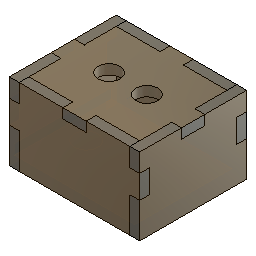
Wooden Preamp Box v5 (Autodesk Fusion 360 design; units mm, degrees)
Autodesk Fusion 360 part; units mm, degrees
note: some values were not read from the file. Chosen so that the rebuilt part matches the saved one: which face or edge a step refers to; a direction.
sketch "Sketch1" plane through (0, 0, 0) normal (1, 0, 0) x (0, 0, -1) in component "Open End"
  line L0 (-29.1465, 0) -> (-29.1465, 19.1516)
  line L1 (-29.1465, 19.1516) -> (-23.8125, 19.1516)
  line L2 (-23.8125, 19.1516) -> (-23.8125, 31.8516)
  line L3 (-23.8125, 31.8516) -> (-29.1465, 31.8516)
  line L4 (-29.1465, 31.8516) -> (-29.1465, 41.9608)
  line L5 (-29.1465, 41.9608) -> (-6.35, 41.9608)
  line L6 (-6.35, 41.9608) -> (-6.35, 36.6268)
  line L7 (-6.35, 36.6268) -> (0, 36.6268)
  line L8 (0, 36.6268) -> (0, 0)
  line L9 (-29.1465, 0) -> (-23.8125, 0)
  line L10 (-23.8125, 0) -> (-23.8125, 3.6576)
  line L11 (-23.8125, 3.6576) -> (-26.4795, 3.6576)
  line L12 (-26.4795, 3.6576) -> (-26.4795, 9.0424)
  line L13 (-26.4795, 9.0424) -> (0, 9.0424)
  line L14 (-29.1465, 25.5016) -> (0, 25.5016) construction
  line L15 (-23.8125, 0) -> (0, 0)
  dimension "d5" = 5.334
  dimension "d6" = 5.334
  dimension "d7" = 5.3848
  dimension "d9" = 2.667
  dimension "d10" = 3.6576
  dimension "d11" = 27.5844
  dimension "d12" = 16.4592
  dimension "d13" = 6.35
  dimension "d14" = 6.35
  dimension "d15" = 23.8125
  dimension "d16" = 6.35
  measures "d7" distance of L11 L13
  measures "d9" distance of L0 L12
  measures "d10" distance of L8.end
  measures "d11" distance of L7 L13
  measures "d12" distance of L5 L14
  measures "d13" distance of L1 L14
  measures "d14" distance of L3 L14
  measures "d15" distance of L2 L8
extrude "Extrude1" add sketch "Sketch1" along normal blind 5.334 contours L0 L1 L2 L3 L4 L5 L6 L7 L8 L9 L10 L11 L12 L13 makes body 1 in component "Open End"
mirror "Mirror1" about plane through (0, 36.6268, 0) normal (0, 0, -1) of bodies 1 makes body 2 in component "Open End"
combine "Combine1" operation add target body 2 tool bodies 1 in component "Open End"
sketch "Sketch1 (2)" plane through (0, 0, 0) normal (1, 0, 0) x (0, 0, -1) in component "Closed End"
  line L0 (-29.1465, 0) -> (-29.1465, 19.1516)
  line L1 (-29.1465, 19.1516) -> (-23.8125, 19.1516)
  line L2 (-23.8125, 19.1516) -> (-23.8125, 31.8516)
  line L3 (-23.8125, 31.8516) -> (-29.1465, 31.8516)
  line L4 (-29.1465, 31.8516) -> (-29.1465, 41.9608)
  line L5 (-29.1465, 41.9608) -> (-6.35, 41.9608)
  line L6 (-6.35, 41.9608) -> (-6.35, 36.6268)
  line L7 (-6.35, 36.6268) -> (0, 36.6268)
  line L8 (0, 36.6268) -> (0, 0)
  line L9 (-29.1465, 0) -> (-23.8125, 0)
  line L10 (-23.8125, 0) -> (-23.8125, 3.6576)
  line L11 (-23.8125, 3.6576) -> (-26.4795, 3.6576)
  line L12 (-26.4795, 3.6576) -> (-26.4795, 9.0424)
  line L13 (-26.4795, 9.0424) -> (0, 9.0424)
  line L14 (-29.1465, 25.5016) -> (0, 25.5016) construction
  line L15 (-23.8125, 0) -> (0, 0)
  dimension "d5_1" = 5.334
  dimension "d6_1" = 5.334
  dimension "d7_1" = 5.3848
  dimension "d9_1" = 2.667
  dimension "d10_1" = 3.6576
  dimension "d11_1" = 27.5844
  dimension "d12_1" = 16.4592
  dimension "d13_1" = 6.35
  dimension "d14_1" = 6.35
  dimension "d15_1" = 23.8125
  dimension "d16_1" = 6.35
  measures "d7_1" distance of L11 L13
  measures "d9_1" distance of L0 L12
  measures "d10_1" distance of L8.end
  measures "d11_1" distance of L7 L13
  measures "d12_1" distance of L5 L14
  measures "d13_1" distance of L1 L14
  measures "d14_1" distance of L3 L14
  measures "d15_1" distance of L2 L8
extrude "Extrude1'" add sketch "Sketch1 (2)" along normal blind 5.334 separate body makes body 3 in component "Closed End"
mirror "Mirror1'" about plane through (0, 9.0424, 0) normal (0, 0, -1) of bodies 3 makes body 4 in component "Closed End"
combine "Combine1'" operation add target body 4 tool bodies 3 in component "Closed End"
sketch "Sketch1 (3)" plane through (0, 0, 0) normal (0, 0, 1) x (1, 0, 0) in component "Front and Back"
  line L0 (0, 41.9608) -> (70.993, 41.9608)
  line L1 (70.993, 41.9608) -> (70.993, 0)
  line L2 (70.993, 0) -> (0, 0)
  line L3 (0, 0) -> (0, 41.9608)
  line L4 (35.4965, 41.9608) -> (35.4965, 0) construction
  line L5 (41.8465, 47.2948) -> (29.1465, 47.2948)
  line L6 (29.1465, 47.2948) -> (29.1465, 36.6268)
  line L7 (29.1465, 36.6268) -> (41.8465, 36.6268)
  line L8 (41.8465, 36.6268) -> (41.8465, 47.2948)
  line L9 (41.8465, 47.2948) -> (29.1465, 36.6268) construction
  line L10 (29.1465, 47.2948) -> (41.8465, 36.6268) construction
  dimension "d27" = 12.7
  dimension "d28" = 10.668
extrude "Extrude1''" add sketch "Sketch1 (3)" against normal blind 5.334 from surface at 29.1465 separate body contours L0 L1 L2 L3 L6 L7 L8 makes body 5 in component "Front and Back"
combine "Combine1''" operation cut target body 5 tool bodies 4 2 body 4 seen with x (1, 0, 0) y (0, 1, 0) z (0, 0, 1) at (65.659, 0, 0) keep tools in component "Front and Back"
extrude "Extrude2" cut 1 faces at (0, 5.4525, 25.5905) along direction (1, 0, 0) through all on bodies 5 bodies 5 in component "Front and Back"
ref_plane "WorkPlane1" through (2.667, 36.9062, 0) normal (0, 0, -1) x (0, -1, 0)
mirror "MirrorComponent1" about plane through (0, 0, 0) normal (0, 0, 1) of bodies 5 makes body 6 in component "Front and Back(Mirror)"
sketch "Sketch1 (4)" plane through (0, 0, 0) normal (0, 1, 0) x (1, 0, 0) in component "Top"
  line L0 (0, 29.1465) -> (70.993, 29.1465)
  line L1 (70.993, 29.1465) -> (70.993, -29.1465)
  line L2 (70.993, -29.1465) -> (0, -29.1465)
  line L3 (0, -29.1465) -> (0, 29.1465)
  line L4 (5.334, -6.35) -> (5.334, -29.1465)
  line L5 (0, 0) -> (70.993, 0) construction
  dimension "d31" = 20.6375
  dimension "d33" = 19.8437
  measures "d33" distance of L4
extrude "Extrude1'''" add sketch "Sketch1 (4)" against normal blind 5.334 from surface at 41.9608 separate body makes body 7 in component "Top"
combine "Combine1'''" operation cut target body 7 tool bodies 4 5 2 6 body 4 seen with x (1, 0, 0) y (0, 1, 0) z (0, 0, 1) at (65.659, 0, 0) keep tools in component "Top"
sketch "Sketch1 (5)" plane through (0, 0, 0) normal (1, 0, 0) x (0, 0, -1) in component "Bottom"
  line L0 (26.4795, 9.0424) -> (-26.4795, 9.0424)
  line L1 (-26.4795, 9.0424) -> (-26.4795, 3.6576)
  line L2 (-26.4795, 3.6576) -> (26.4795, 3.6576)
  line L3 (26.4795, 3.6576) -> (26.4795, 9.0424)
extrude "Extrude1''''" add sketch "Sketch1 (5)" along normal blind 65.659 separate body makes body 8 in component "Bottom"
hole "Hole1" at (25.1777, 0, 0) at (45.8153, 0, 0) direction (0, 1, 0) diameter 11.9062 depth 41.9608 tip angle 118 bodies 7 in component "Top"
sketch "Sketch2" plane through (0, 0, 0) normal (0, 1, 0) x (1, 0, 0) in component "Bottom"
  line L0 (0, 0) -> (70.993, 0)
  dimension "d37" = 12.7
  measures "d37" distance of L0.start
hole "Hole1'" at (12.7, 0, 0) direction (0, 1, 0) diameter 12.7 depth 41.9608 tip angle 118 bodies 8 in component "Bottom"
sketch "dxf top" plane through (0, 41.9608, 0) normal (0, 1, 0) x (-1, 0, 0)
  circle A0 centre (-25.1777, 0) radius 5.9531
  circle A1 centre (-45.8153, 0) radius 5.9531
  line L0 (-29.1465, -23.8125) -> (-5.334, -23.8125)
  line L1 (-5.334, -23.8125) -> (-5.334, -6.35)
  line L2 (-5.334, -6.35) -> (0, -6.35)
  line L3 (0, -6.35) -> (0, 6.35)
  line L4 (0, 6.35) -> (-5.334, 6.35)
  line L5 (-5.334, 6.35) -> (-5.334, 23.8125)
  line L6 (-5.334, 23.8125) -> (-29.1465, 23.8125)
  line L7 (-29.1465, 23.8125) -> (-29.1465, 29.1465)
  line L8 (-29.1465, 29.1465) -> (-41.8465, 29.1465)
  line L9 (-41.8465, 29.1465) -> (-41.8465, 23.8125)
  line L10 (-41.8465, 23.8125) -> (-65.659, 23.8125)
  line L11 (-65.659, 23.8125) -> (-65.659, 6.35)
  line L12 (-65.659, 6.35) -> (-70.993, 6.35)
  line L13 (-70.993, 6.35) -> (-70.993, -6.35)
  line L14 (-70.993, -6.35) -> (-65.659, -6.35)
  line L15 (-65.659, -6.35) -> (-65.659, -23.8125)
  line L16 (-65.659, -23.8125) -> (-41.8465, -23.8125)
  line L17 (-41.8465, -23.8125) -> (-41.8465, -29.1465)
  line L18 (-41.8465, -29.1465) -> (-29.1465, -29.1465)
  line L19 (-29.1465, -29.1465) -> (-29.1465, -23.8125)
sketch "dxf open side" plane through (0, 0, 0) normal (-1, 0, 0) x (0, 0, 1)
  line L0 (-29.1465, 0) -> (-23.8125, 0)
  line L1 (-23.8125, 0) -> (-23.8125, 3.6576)
  line L2 (-23.8125, 3.6576) -> (-26.4795, 3.6576)
  line L3 (-26.4795, 3.6576) -> (-26.4795, 9.0424)
  line L4 (-26.4795, 9.0424) -> (26.4795, 9.0424)
  line L5 (26.4795, 9.0424) -> (26.4795, 3.6576)
  line L6 (26.4795, 3.6576) -> (23.8125, 3.6576)
  line L7 (23.8125, 3.6576) -> (23.8125, 0)
  line L8 (23.8125, 0) -> (29.1465, 0)
  line L9 (29.1465, 0) -> (29.1465, 19.1516)
  line L10 (29.1465, 19.1516) -> (23.8125, 19.1516)
  line L11 (23.8125, 19.1516) -> (23.8125, 31.8516)
  line L12 (23.8125, 31.8516) -> (29.1465, 31.8516)
  line L13 (29.1465, 31.8516) -> (29.1465, 41.9608)
  line L14 (29.1465, 41.9608) -> (6.35, 41.9608)
  line L15 (6.35, 41.9608) -> (6.35, 36.6268)
  line L16 (6.35, 36.6268) -> (-6.35, 36.6268)
  line L17 (-6.35, 36.6268) -> (-6.35, 41.9608)
  line L18 (-6.35, 41.9608) -> (-29.1465, 41.9608)
  line L19 (-29.1465, 41.9608) -> (-29.1465, 31.8516)
  line L20 (-29.1465, 31.8516) -> (-23.8125, 31.8516)
  line L21 (-23.8125, 31.8516) -> (-23.8125, 19.1516)
  line L22 (-23.8125, 19.1516) -> (-29.1465, 19.1516)
  line L23 (-29.1465, 19.1516) -> (-29.1465, 0)
sketch "dxf front and back" plane through (0, 0, 29.1465) normal (0, 0, 1) x (1, 0, 0)
  line L0 (5.334, 19.1516) -> (5.334, 0)
  line L1 (5.334, 0) -> (65.659, 0)
  line L2 (65.659, 0) -> (65.659, 19.1516)
  line L3 (65.659, 19.1516) -> (70.993, 19.1516)
  line L4 (70.993, 19.1516) -> (70.993, 31.8516)
  line L5 (70.993, 31.8516) -> (65.659, 31.8516)
  line L6 (65.659, 31.8516) -> (65.659, 41.9608)
  line L7 (65.659, 41.9608) -> (41.8465, 41.9608)
  line L8 (41.8465, 41.9608) -> (41.8465, 36.6268)
  line L9 (41.8465, 36.6268) -> (29.1465, 36.6268)
  line L10 (29.1465, 36.6268) -> (29.1465, 41.9608)
  line L11 (29.1465, 41.9608) -> (5.334, 41.9608)
  line L12 (5.334, 41.9608) -> (5.334, 31.8516)
  line L13 (5.334, 31.8516) -> (0, 31.8516)
  line L14 (0, 31.8516) -> (0, 19.1516)
  line L15 (0, 19.1516) -> (5.334, 19.1516)
sketch "dxf closed side" plane through (70.993, 0, 0) normal (1, 0, 0) x (0, 0, -1)
  line L0 (-29.1465, 0) -> (29.1465, 0)
  line L1 (29.1465, 0) -> (29.1465, 19.1516)
  line L2 (29.1465, 19.1516) -> (23.8125, 19.1516)
  line L3 (23.8125, 19.1516) -> (23.8125, 31.8516)
  line L4 (23.8125, 31.8516) -> (29.1465, 31.8516)
  line L5 (29.1465, 31.8516) -> (29.1465, 41.9608)
  line L6 (29.1465, 41.9608) -> (6.35, 41.9608)
  line L7 (6.35, 41.9608) -> (6.35, 36.6268)
  line L8 (6.35, 36.6268) -> (-6.35, 36.6268)
  line L9 (-6.35, 36.6268) -> (-6.35, 41.9608)
  line L10 (-6.35, 41.9608) -> (-29.1465, 41.9608)
  line L11 (-29.1465, 41.9608) -> (-29.1465, 31.8516)
  line L12 (-29.1465, 31.8516) -> (-23.8125, 31.8516)
  line L13 (-23.8125, 31.8516) -> (-23.8125, 19.1516)
  line L14 (-23.8125, 19.1516) -> (-29.1465, 19.1516)
  line L15 (-29.1465, 19.1516) -> (-29.1465, 0)
sketch "dxf bottom" plane through (0, 3.6576, 0) normal (0, -1, 0) x (1, 0, 0)
  circle A0 centre (12.7, 0) radius 6.35
  line L0 (0, 26.4795) -> (0, -26.4795)
  line L1 (0, -26.4795) -> (65.659, -26.4795)
  line L2 (65.659, -26.4795) -> (65.659, 26.4795)
  line L3 (65.659, 26.4795) -> (0, 26.4795)
component "Open End" placed x (1, 0, 0) y (0, 1, 0) z (0, 0, 1) at (0, 0, 0)
component "Closed End" placed x (1, 0, 0) y (0, 1, 0) z (0, 0, 1) at (65.659, 0, 0)
component "Front and Back" placed x (1, 0, 0) y (0, 1, 0) z (0, 0, 1) at (0, 0, 0)
component "Top" placed x (1, 0, 0) y (0, 1, 0) z (0, 0, 1) at (0, 0, 0)
component "Front and Back(Mirror)" placed x (1, 0, 0) y (0, 1, 0) z (0, 0, 1) at (0, 0, 0)
component "Bottom" placed x (1, 0, 0) y (0, 1, 0) z (0, 0, 1) at (0, 0, 0)
equation "thickness = 0.210 in" comment "Birch Plywood"
equation "width_inside = 2.375 in"
equation "depth_inside = 1.875 in"
equation "height_inside = 1 in + 0.086 in"
equation "d5 = thickness"
equation "d6 = thickness"
equation "d7 = thickness + 0.002 in"
equation "d9 = thickness / 2"
equation "d10 = thickness - 0.066 in"
equation "d11 = height_inside"
equation "d12 = ( height_inside + thickness ) / 2"
equation "d15 = depth_inside / 2"
equation "d17 = thickness"
equation "d5_1 = thickness"
equation "d6_1 = thickness"
equation "d7_1 = thickness + 0.002 in"
equation "d9_1 = thickness / 2"
equation "d10_1 = thickness - 0.066 in"
equation "d11_1 = height_inside"
equation "d12_1 = ( height_inside + thickness ) / 2"
equation "d15_1 = depth_inside / 2"
equation "d17_1 = thickness"
equation "d21 = -thickness"
equation "d25 = -thickness"
equation "d28 = thickness * 2"
equation "d31 = ( 13 / 16 ) * 1 in"
equation "d33 = width_inside / 2 - d31 / 2"
equation "d35 = ( 15 / 32 ) * 1 in"
